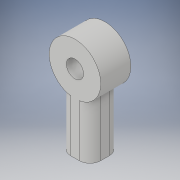
# Autodesk Inventor part: Eye Bolt
Saved by Autodesk Inventor 2019.4 (Build 234330000, 330)
## iProperties
Created: 2020-01-29
Part Number: Eye Bolt
Material: Generic
Document SubType Name: Modeling
Designer: admin
Density: 1 g/cm^3
Appearance: Default
Author: admin
Autodesk Inventor part; units mm, degrees
ref_plane "YZ Plane" through (0, 0, 0) normal (1, 0, 0) x (0, 1, 0)
ref_plane "XZ Plane" through (0, 0, 0) normal (0, 1, 0) x (-1, 0, 0)
ref_plane "XY Plane" through (0, 0, 0) normal (0, 0, 1) x (1, 0, 0)
sketch "Sketch1" plane through (0, 0, 0) normal (0, 0, 1) x (1, 0, 0)
  circle A0 centre (0, 0) radius 4
  arc A1 (7, -9.7468) -> (-7, -9.7468) centre (0, 0) ccw
  line L0 (-7, -9.7468) -> (-7, -36)
  line L1 (-7, -36) -> (7, -36)
  line L2 (7, -36) -> (7, -9.7468)
  arc A2 (-7, -9.7468) -> (7, -9.7468) centre (0, 0) ccw construction
  dimension "d0" = 8
  dimension "d1" = 24
  dimension "d2" = 14
  dimension "d3" = 36
  constraints: 6 end point, 4 point on circle, 3 centre point, 2 coincident, 2 perpendicular, 1 parallel, 1 vertical
  measures "d0" diameter of A0
  measures "d1" diameter of A1
  measures "d2" distance of L0.end L1.end
  measures "d3" distance from line of L1 A0.centre
extrude "Extrusion1" add sketch "Sketch1" along normal blind 14
sketch "Sketch2" plane through (-7, -36, 0) normal (0, -1, 0) x (1, 0, 0)
  circle A0 centre (7, 7) radius 4.4
  line L0 (7, 7) -> (7, 0) construction
  line L1 (7, 7) -> (14, 7) construction
  line L2 (14, 0) -> (14, 14) projected
  dimension "d6" = 8.8
  constraints: 4 end point, 1 centre point, 1 midpoint, 1 perpendicular, 1 vertical
  measures "d6" diameter of A0
extrude "Extrusion2" cut sketch "Sketch2" against normal blind 30
fillet "Fillet1" radius 5 4 edges at (7, -22.8734, 14) (7, -22.8734, 0) (-7, -22.8734, 14) (-7, -22.8734, 0)
body "Solid1"
